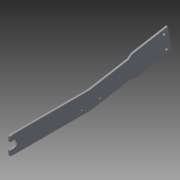
# Autodesk Inventor part: Arm_Link_1
Saved by Autodesk Inventor 2013 (Build 170138000, 138)
## iProperties
Created: 2014-05-15
Part Number: Arm_Link_1
Material: 一般
Document SubType Name: Modeling
Designer: andou
Density: 1 g/cm^3
Author: andou
Autodesk Inventor part; units mm, degrees
ref_plane "YZ Plane" through (0, 0, 0) normal (1, 0, 0) x (0, 1, 0)
ref_plane "XZ Plane" through (0, 0, 0) normal (0, 1, 0) x (-1, 0, 0)
ref_plane "XY Plane" through (0, 0, 0) normal (0, 0, 1) x (1, 0, 0)
sketch "スケッチ2" plane through (0, 0, 0) normal (1, 0, 0) x (0, 1, 0)
  line L0 (0, 0) -> (-84.4498, 0)
  line L1 (-84.4498, -20) -> (1.7498, -20)
  line L2 (0, 0) -> (83.1668, 14.6646)
  line L3 (86.6398, -5.0316) -> (1.7498, -20)
  arc A0 (87.251, 14.537) -> (83.1668, 14.6646) centre (84.9033, 4.8165) ccw
  arc A1 (86.6398, -5.0316) -> (90.434, -3.5148) centre (84.9033, 4.8165) ccw
  arc A2 (-88.4498, -19.1652) -> (-84.4498, -20) centre (-84.4498, -10) ccw
  arc A3 (-84.4498, 0) -> (-88.4498, -0.8348) centre (-84.4498, -10) ccw
  arc A4 (-84.4498, -14) -> (-84.4498, -6) centre (-84.4498, -10) ccw
  line L4 (-84.4498, -6) -> (-88.4498, -6)
  line L5 (-84.4498, -14) -> (-88.4498, -14)
  line L6 (-88.4498, -0.8348) -> (-88.4498, -6)
  line L7 (-88.4498, -14) -> (-88.4498, -19.1652)
  line L8 (87.251, 14.537) -> (88.1479, 9.4503)
  line L9 (89.5371, 1.5718) -> (90.434, -3.5148)
  line L10 (1.7498, -20) -> (0, 0)
  line L11 (88.1479, 9.4503) -> (89.5371, 1.5718)
  dimension "d21" = 20
  dimension "d22" = 10
  dimension "d23" = 170
  dimension "d25" = 10
  dimension "d27" = 10
  dimension "d31" = 8
  dimension "d33" = 4
  dimension "d35" = 4
  dimension "d36" = 170
  constraints: 24 end point, 10 point on circle, 8 perpendicular, 5 centre point, 4 equal length, 3 equal radius, 2 parallel, 2 tangent, 1 coincident, 1 collinear, 1 horizontal
  measures "d21" distance between parallel lines of L0 L1
  measures "d22" distance from line of L0 A2.centre
  measures "d23" angle of L0 L2
  measures "d25" distance from line of L3 A0.centre
  measures "d27" radius of A3
  measures "d31" diameter of A4
  measures "d33" distance from line of L6 A2.centre
  measures "d35" distance from line of L8 L2.end
  measures "d36" distance of A2.centre A0.centre
extrude "押し出し1" add sketch "スケッチ2" along normal blind 2
sketch "スケッチ4" plane through (0, 0, 0) normal (-1, 0, 0) x (0, 0, 1)
  line L0 (-20, 1.7498) -> (-5.0316, 86.6398) projected
  line L1 (-20, -84.4498) -> (-20, 1.7498) projected
  circle A0 centre (-15, -8.7259) radius 1
  circle A1 centre (-13.2569, 11.198) radius 1
  line L2 (-15, -8.7259) -> (-13.2569, 11.198)
  dimension "d57" = 2
  dimension "d59" = 20
  dimension "d60" = 175
  dimension "d61" = 5
  dimension "d62" = 5
  constraints: 2 centre point, 2 end point, 1 equal radius
  measures "d57" diameter of A0
  measures "d59" distance of L2.start L2.end
  measures "d60" angle of L1 L2
  measures "d61" distance from line of L1 L2.start
  measures "d62" distance from line of L0 L2.end
hole "穴2" at (0, -8.7259, -15) at (0, 11.198, -13.2569) direction (1, 0, 0) diameter 1.6 end through all
sketch "スケッチ6" plane through (2, 0, 0) normal (1, 0, 0) x (0, 0, -1)
  line L0 (20, 1.7498) -> (5.0316, 86.6398) projected
  arc A0 (5.0316, 86.6398) -> (3.5148, 90.434) centre (-4.8165, 84.9033) ccw projected
  line L1 (3.5148, 90.434) -> (-14.537, 87.251) projected
  arc A1 (-14.537, 87.251) -> (-14.6646, 83.1668) centre (-4.8165, 84.9033) ccw projected
  line L2 (-14.6646, 83.1668) -> (0, 0) projected
  line L3 (-7.6613, 43.4494) -> (-10.8752, 47.2796)
  line L4 (-14.537, 87.251) -> (-17.8212, 86.6719)
  line L5 (-17.8212, 86.6719) -> (-10.8752, 47.2796)
  line L6 (3.5148, 90.434) -> (6.799, 91.0131)
  line L7 (6.799, 91.0131) -> (13.745, 51.6208)
  line L8 (13.745, 51.6208) -> (12.0349, 46.9224)
  dimension "d75" = 150
  dimension "d76" = 150
  dimension "d77" = 2.5
  dimension "d78" = 2.5
  dimension "d79" = 40
  constraints: 12 end point, 3 parallel, 2 collinear, 2 point on line
  measures "d75" angle of L2 L3
  measures "d76" angle of L0 L8
  measures "d77" distance between parallel lines of L0 L7
  measures "d78" distance between parallel lines of L2 L5
  measures "d79" distance of L4.end L3.end
extrude "押し出し2" add sketch "スケッチ6" against normal blind 2
sketch "スケッチ5" plane through (2, 0, 0) normal (1, 0, 0) x (0, 0, -1)
  line L0 (3.5148, 90.434) -> (-14.537, 87.251) projected
  line L1 (-14.6646, 83.1668) -> (0, 0) projected
  circle A0 centre (-12.5213, 82.5293) radius 1.5
  circle A1 centre (3.2356, 85.3077) radius 1.5
  line L2 (-10.8752, 47.2796) -> (-17.8212, 86.6719) projected
  line L3 (-17.8212, 86.6719) -> (6.799, 91.0131) projected
  line L4 (6.799, 91.0131) -> (13.745, 51.6208) projected
  line L5 (13.745, 51.6208) -> (12.0349, 46.9224) projected
  line L6 (12.0349, 46.9224) -> (20, 1.7498) projected
  line L7 (20, 1.7498) -> (20, -84.4498) projected
  arc A2 (19.1652, -88.4498) -> (20, -84.4498) centre (10, -84.4498) ccw projected
  line L8 (19.1652, -88.4498) -> (14, -88.4498) projected
  line L9 (14, -88.4498) -> (14, -84.4498) projected
  arc A3 (14, -84.4498) -> (6, -84.4498) centre (10, -84.4498) ccw projected
  line L10 (6, -84.4498) -> (6, -88.4498) projected
  line L11 (6, -88.4498) -> (0.8348, -88.4498) projected
  arc A4 (0, -84.4498) -> (0.8348, -88.4498) centre (10, -84.4498) ccw projected
  line L12 (0, -84.4498) -> (0, 0) projected
  line L13 (0, 0) -> (-7.6613, 43.4494) projected
  line L14 (-7.6613, 43.4494) -> (-10.8752, 47.2796) projected
  circle A5 centre (15, -8.7259) radius 0.8 projected
  circle A6 centre (13.2569, 11.198) radius 0.8 projected
  dimension "d70" = 5
  dimension "d71" = 5
  dimension "d72" = 3
  dimension "d73" = 16
  dimension "d74" = 2
  constraints: 2 centre point, 1 equal radius
  measures "d70" distance from line of L0 A0.centre
  measures "d71" distance from line of L0 A1.centre
  measures "d72" diameter of A1
  measures "d73" distance of A1.centre A0.centre
  measures "d74" distance from line of L1 A0.centre
hole "穴3" at (2, 82.5293, 12.5213) at (2, 85.3077, -3.2356) direction (-1, 0, 0) diameter 3 end through all
